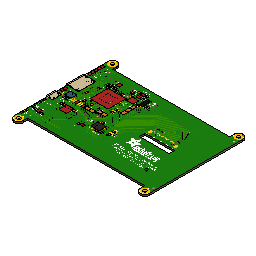
Adafruit 5in HDMI Backpack v2 (Autodesk Fusion 360 design; units mm, degrees)
part number: 47151-0001
part number: TFP401
part number: 1uF
part number: Ferrite
part number: MOUNTINGHOLE3.0
part number: FIDUCIAL""
part number: FAN5333BSX
part number: LT1117(3V3)
part number: MicroUSB
part number: AR1100
part number: 12MHz
part number: 33
part number: Blue
part number: 15uH
part number: MBR0540
part number: MM3Z24VT1G
part number: BSS138
part number: TFTLCD-KD50G21-40NT-A1
part number: 1N4148
part number: 100uF/6V
Autodesk Fusion 360 part; units mm, degrees
sketch "sketch 301" plane through (0, 0, 0) normal (0, 0, 1) x (1, 0, 0)
  line L0 (8, 0) -> (112.7, 0)
  line L1 (112.7, 0) -> (112.7, -4)
  arc A0 (112.7, -4) -> (116.7, -8) centre (116.7, -4) ccw
  arc A1 (116.7, -8) -> (120.7, -4) centre (116.7, -4) ccw
  line L2 (120.7, -4) -> (120.7, 79.8)
  arc A2 (120.7, 79.8) -> (116.7, 83.8) centre (116.7, 79.8) ccw
  arc A3 (116.7, 83.8) -> (112.7, 79.9) centre (116.65, 79.85) ccw
  line L3 (112.7, 79.9) -> (112.7, 75.8)
  line L4 (112.7, 75.8) -> (8, 75.8)
  line L5 (8, 75.8) -> (8, 79.8)
  arc A4 (8, 79.8) -> (4, 83.8) centre (4, 79.8) ccw
  arc A5 (4, 83.8) -> (0, 79.8) centre (4, 79.8) ccw
  line L6 (0, 79.8) -> (0, -4)
  arc A6 (0, -4) -> (4, -8) centre (4, -4) ccw
  arc A7 (4, -8) -> (8, -4) centre (4, -4) ccw
  line L7 (8, -4) -> (8, 0)
  line L8 (98.778, 35.73) -> (98.778, 40.752)
  line L9 (98.778, 40.752) -> (72.108, 40.752)
  line L10 (72.108, 40.752) -> (72.108, 35.73)
  line L11 (72.108, 35.73) -> (98.778, 35.73)
  arc A8 (7.15, 58.25) -> (7.6, 57.8) centre (7.6, 58.25) ccw
  arc A9 (7.6, 58.7) -> (7.15, 58.25) centre (7.6, 58.25) ccw
  line L12 (7.6, 58.7) -> (9.4, 58.7)
  arc A10 (9.85, 58.25) -> (9.4, 58.7) centre (9.4, 58.25) ccw
  arc A11 (9.4, 57.8) -> (9.85, 58.25) centre (9.4, 58.25) ccw
  line L13 (9.4, 57.8) -> (7.6, 57.8)
  arc A12 (2.13, 44.2) -> (1.68, 43.75) centre (2.13, 43.75) ccw
  line L14 (2.13, 44.2) -> (2.93, 44.2)
  arc A13 (3.38, 43.75) -> (2.93, 44.2) centre (2.93, 43.75) ccw
  arc A14 (2.93, 43.3) -> (3.38, 43.75) centre (2.93, 43.75) ccw
  line L15 (2.93, 43.3) -> (2.13, 43.3)
  arc A15 (1.68, 43.75) -> (2.13, 43.3) centre (2.13, 43.75) ccw
  line L16 (7.6, 43.3) -> (9.4, 43.3)
  arc A16 (9.4, 43.3) -> (9.85, 43.75) centre (9.4, 43.75) ccw
  arc A17 (9.85, 43.75) -> (9.4, 44.2) centre (9.4, 43.75) ccw
  line L17 (9.4, 44.2) -> (7.6, 44.2)
  arc A18 (7.6, 44.2) -> (7.15, 43.75) centre (7.6, 43.75) ccw
  arc A19 (7.15, 43.75) -> (7.6, 43.3) centre (7.6, 43.75) ccw
  arc A20 (2.13, 58.7) -> (1.68, 58.25) centre (2.13, 58.25) ccw
  line L18 (2.13, 58.7) -> (2.93, 58.7)
  arc A21 (3.38, 58.25) -> (2.93, 58.7) centre (2.93, 58.25) ccw
  arc A22 (2.93, 57.8) -> (3.38, 58.25) centre (2.93, 58.25) ccw
  line L19 (2.93, 57.8) -> (2.13, 57.8)
  arc A23 (1.68, 58.25) -> (2.13, 57.8) centre (2.13, 58.25) ccw
  arc A24 (2.4, 33.2) -> (2.15, 33.5) centre (2.125, 33.225) ccw
  arc A25 (2.15, 32.9) -> (2.4, 33.2) centre (2.125, 33.175) ccw
  line L20 (2.15, 32.9) -> (1.55, 32.9)
  arc A26 (1.3, 33.2) -> (1.55, 32.9) centre (1.575, 33.175) ccw
  arc A27 (1.55, 33.5) -> (1.3, 33.2) centre (1.575, 33.225) ccw
  line L21 (1.55, 33.5) -> (2.15, 33.5)
  arc A28 (2.15, 25.7) -> (2.4, 26) centre (2.125, 25.975) ccw
  line L22 (2.15, 25.7) -> (1.55, 25.7)
  arc A29 (1.3, 26) -> (1.55, 25.7) centre (1.575, 25.975) ccw
  arc A30 (1.55, 26.3) -> (1.3, 26) centre (1.575, 26.025) ccw
  line L23 (1.55, 26.3) -> (2.15, 26.3)
  arc A31 (2.4, 26) -> (2.15, 26.3) centre (2.125, 26.025) ccw
extrude "Board" add sketch "sketch 301" along normal blind 1.57 makes body 1 in component "Board"
sketch "sketch 2066" plane through (0, 0, 0) normal (0, 0, 1) x (1, 0, 0)
  line L0 (-7.7, -10.31) -> (7.7, -10.31)
  line L1 (7.7, -10.31) -> (7.7, 1)
  line L2 (7.7, 1) -> (-7.7, 1)
  line L3 (-7.7, 1) -> (-7.7, -10.31)
extrude "HDMI_MOLEX_47151-0001_DIMLAYER" add sketch "sketch 2066" along normal blind 0.1 separate body makes body 2 in component "HDMI_MOLEX_47151-0001_DIMLAYER"
sketch "sketch 2197" plane through (0, 0, 0) normal (0, 0, 1) x (1, 0, 0)
  line L0 (-8.12, -8.12) -> (8, -8.12)
  line L1 (8, -8.12) -> (8, 8)
  line L2 (8, 8) -> (-8.12, 8)
  line L3 (-8.12, 8) -> (-8.12, -8.12)
extrude "S-PQFP-G100" add sketch "sketch 2197" along normal blind 0.1 separate body makes body 3 in component "S-PQFP-G100"
sketch "sketch 2584" plane through (0, 0, 0) normal (0, 0, 1) x (1, 0, 0)
  line L0 (-1.092, -0.724) -> (1.106, -0.724)
  line L1 (1.106, -0.724) -> (1.106, 0.726)
  line L2 (1.106, 0.726) -> (-1.092, 0.726)
  line L3 (-1.092, 0.726) -> (-1.092, -0.724)
extrude "0805-NO" add sketch "sketch 2584" along normal blind 0.1 separate body makes body 4 in component "0805-NO"
sketch "sketch 2803" plane through (0, 0, 0) normal (0, 0, 1) x (1, 0, 0)
  line L0 (-1, -0.65) -> (1, -0.65)
  line L1 (1, -0.65) -> (1, 0.65)
  line L2 (1, 0.65) -> (-1, 0.65)
  line L3 (-1, 0.65) -> (-1, -0.65)
extrude "_0805MP" add sketch "sketch 2803" along normal blind 0.1 separate body makes body 5 in component "_0805MP"
sketch "sketch 2942" plane through (0, 0, 0) normal (0, 0, 1) x (1, 0, 0)
  line L0 (-1.651, -1.016) -> (1.651, -1.016)
  line L1 (1.651, -1.016) -> (1.651, 1.016)
  line L2 (1.651, 1.016) -> (-1.651, 1.016)
  line L3 (-1.651, 1.016) -> (-1.651, -1.016)
extrude "SOLDERJUMPER_ARROW_NOPASTE" add sketch "sketch 2942" along normal blind 0.1 separate body makes body 6 in component "SOLDERJUMPER_ARROW_NOPASTE"
sketch "sketch 3097" plane through (0, 0, 0) normal (0, 0, 1) x (1, 0, 0)
  line L0 (-3.429, -3.429) -> (3.429, -3.429)
  line L1 (3.429, -3.429) -> (3.429, 3.429)
  line L2 (3.429, 3.429) -> (-3.429, 3.429)
  line L3 (-3.429, 3.429) -> (-3.429, -3.429)
extrude "MOUNTINGHOLE_3.0_PLATED" add sketch "sketch 3097" along normal blind 0.1 separate body makes body 7 in component "MOUNTINGHOLE_3.0_PLATED"
sketch "sketch 3268" plane through (0, 0, 0) normal (0, 0, 1) x (1, 0, 0)
  line L0 (-0.75, -0.75) -> (0.75, -0.75)
  line L1 (0.75, -0.75) -> (0.75, 0.75)
  line L2 (0.75, 0.75) -> (-0.75, 0.75)
  line L3 (-0.75, 0.75) -> (-0.75, -0.75)
extrude "FIDUCIAL_1MM" add sketch "sketch 3268" along normal blind 0.1 separate body makes body 8 in component "FIDUCIAL_1MM"
sketch "sketch 3407" plane through (0, 0, 0) normal (0, 0, 1) x (1, 0, 0)
  line L0 (-1.65, -1.5) -> (1.65, -1.5)
  line L1 (1.65, -1.5) -> (1.65, 1.5)
  line L2 (1.65, 1.5) -> (-1.65, 1.5)
  line L3 (-1.65, 1.5) -> (-1.65, -1.5)
extrude "SOT23-5" add sketch "sketch 3407" along normal blind 0.1 separate body makes body 9 in component "SOT23-5"
sketch "sketch 3538" plane through (0, 0, 0) normal (0, 0, 1) x (1, 0, 0)
  line L0 (-3.35, -3.45) -> (3.35, -3.45)
  line L1 (3.35, -3.45) -> (3.35, 3.45)
  line L2 (3.35, 3.45) -> (-3.35, 3.45)
  line L3 (-3.35, 3.45) -> (-3.35, -3.45)
extrude "SOT223-R" add sketch "sketch 3538" along normal blind 0.1 separate body makes body 10 in component "SOT223-R"
sketch "sketch 3669" plane through (0, 0, 0) normal (0, 0, 1) x (1, 0, 0)
  line L0 (-3.975, -4.9) -> (4.35, -4.9)
  line L1 (4.35, -4.9) -> (4.35, 1.25)
  line L2 (4.35, 1.25) -> (-3.975, 1.25)
  line L3 (-3.975, 1.25) -> (-3.975, -4.9)
extrude "4UCONN_20329" add sketch "sketch 3669" along normal blind 0.1 separate body makes body 11 in component "4UCONN_20329"
sketch "sketch 3800" plane through (0, 0, 0) normal (0, 0, 1) x (1, 0, 0)
  line L0 (-3.165, -3.821) -> (3.165, -3.821)
  line L1 (3.165, -3.821) -> (3.165, 3.821)
  line L2 (3.165, 3.821) -> (-3.165, 3.821)
  line L3 (-3.165, 3.821) -> (-3.165, -3.821)
extrude "TSSOP20-5.3MMBODY" add sketch "sketch 3800" along normal blind 0.1 separate body makes body 12 in component "TSSOP20-5.3MMBODY"
sketch "sketch 3931" plane through (0, 0, 0) normal (0, 0, 1) x (1, 0, 0)
  line L0 (-1.8, -0.65) -> (1.8, -0.65)
  line L1 (1.8, -0.65) -> (1.8, 0.65)
  line L2 (1.8, 0.65) -> (-1.8, 0.65)
  line L3 (-1.8, 0.65) -> (-1.8, -0.65)
extrude "RESONATOR-SMD" add sketch "sketch 3931" along normal blind 0.1 separate body makes body 13 in component "RESONATOR-SMD"
sketch "sketch 4110" plane through (0, 0, 0) normal (0, 0, 1) x (1, 0, 0)
  line L0 (-1.9, -1.4) -> (1.9, -1.4)
  line L1 (1.9, -1.4) -> (1.9, 1.4)
  line L2 (1.9, 1.4) -> (-1.9, 1.4)
  line L3 (-1.9, 1.4) -> (-1.9, -1.4)
extrude "RESPACK_4X0603" add sketch "sketch 4110" along normal blind 0.1 separate body makes body 14 in component "RESPACK_4X0603"
sketch "sketch 4257" plane through (0, 0, 0) normal (0, 0, 1) x (1, 0, 0)
  line L0 (-0.625, -1.3334) -> (0.625, -1.3334)
  line L1 (0.625, -1.3334) -> (0.625, 1.3334)
  line L2 (0.625, 1.3334) -> (-0.625, 1.3334)
  line L3 (-0.625, 1.3334) -> (-0.625, -1.3334)
extrude "CHIPLED_0805_NOOUTLINE" add sketch "sketch 4257" along normal blind 0.1 separate body makes body 15 in component "CHIPLED_0805_NOOUTLINE"
sketch "sketch 4388" plane through (0, 0, 0) normal (0, 0, 1) x (1, 0, 0)
  line L0 (-2.938, -2.6) -> (2.938, -2.6)
  line L1 (2.938, -2.6) -> (2.938, 2.6)
  line L2 (2.938, 2.6) -> (-2.938, 2.6)
  line L3 (-2.938, 2.6) -> (-2.938, -2.6)
extrude "INDUCTOR_5X5MM_NR5040_NOTHERMALS" add sketch "sketch 4388" along normal blind 0.1 separate body makes body 16 in component "INDUCTOR_5X5MM_NR5040_NOTHERMALS"
sketch "sketch 4519" plane through (0, 0, 0) normal (0, 0, 1) x (1, 0, 0)
  line L0 (-1.723, -0.7) -> (1.723, -0.7)
  line L1 (1.723, -0.7) -> (1.723, 0.7)
  line L2 (1.723, 0.7) -> (-1.723, 0.7)
  line L3 (-1.723, 0.7) -> (-1.723, -0.7)
extrude "SOD-123" add sketch "sketch 4519" along normal blind 0.1 separate body makes body 17 in component "SOD-123"
sketch "sketch 4650" plane through (0, 0, 0) normal (0, 0, 1) x (1, 0, 0)
  line L0 (-3.889, -1.6) -> (3.916, -1.6)
  line L1 (3.916, -1.6) -> (3.916, 1.6)
  line L2 (3.916, 1.6) -> (-3.889, 1.6)
  line L3 (-3.889, 1.6) -> (-3.889, -1.6)
extrude "SMADIODE" add sketch "sketch 4650" along normal blind 0.1 separate body makes body 18 in component "SMADIODE"
sketch "sketch 4781" plane through (0, 0, 0) normal (0, 0, 1) x (1, 0, 0)
  line L0 (-1.672, -1.295) -> (1.672, -1.295)
  line L1 (1.672, -1.295) -> (1.672, 1.295)
  line L2 (1.672, 1.295) -> (-1.672, 1.295)
  line L3 (-1.672, 1.295) -> (-1.672, -1.295)
extrude "SOT23-WIDE" add sketch "sketch 4781" along normal blind 0.1 separate body makes body 19 in component "SOT23-WIDE"
sketch "sketch 4912" plane through (0, 0, 0) normal (0, 0, 1) x (1, 0, 0)
  line L0 (0, 0) -> (120.7, 0)
  line L1 (120.7, 0) -> (120.7, 75.8)
  line L2 (120.7, 75.8) -> (0, 75.8)
  line L3 (0, 75.8) -> (0, 0)
extrude "TFTLCD-KD50G21-40NT-A1" add sketch "sketch 4912" along normal blind 0.1 separate body makes body 20 in component "TFTLCD-KD50G21-40NT-A1"
sketch "sketch 5091" plane through (0, 0, 0) normal (0, 0, 1) x (1, 0, 0)
  line L0 (-1.2, -1.2) -> (1.2, -1.2)
  line L1 (1.2, -1.2) -> (1.2, 1.2)
  line L2 (1.2, 1.2) -> (-1.2, 1.2)
  line L3 (-1.2, 1.2) -> (-1.2, -1.2)
extrude "1X01_SMD_MASKHELD_2X2MM" add sketch "sketch 5091" along normal blind 0.1 separate body makes body 21 in component "1X01_SMD_MASKHELD_2X2MM"
sketch "sketch 5230" plane through (0, 0, 0) normal (0, 0, 1) x (1, 0, 0)
  line L0 (-1.651, -1.016) -> (1.651, -1.016)
  line L1 (1.651, -1.016) -> (1.651, 1.016)
  line L2 (1.651, 1.016) -> (-1.651, 1.016)
  line L3 (-1.651, 1.016) -> (-1.651, -1.016)
extrude "SOLDERJUMPER_CLOSEDWIRE" add sketch "sketch 5230" along normal blind 0.1 separate body makes body 22 in component "SOLDERJUMPER_CLOSEDWIRE"
sketch "sketch 5361" plane through (0, 0, 0) normal (0, 0, 1) x (1, 0, 0)
  line L0 (-1, -0.7) -> (1, -0.7)
  line L1 (1, -0.7) -> (1, 0.7)
  line L2 (1, 0.7) -> (-1, 0.7)
  line L3 (-1, 0.7) -> (-1, -0.7)
extrude "SOD-323" add sketch "sketch 5361" along normal blind 0.1 separate body makes body 23 in component "SOD-323"
sketch "sketch 5492" plane through (0, 0, 0) normal (0, 0, 1) x (1, 0, 0)
  line L0 (-2.95, -2.6) -> (2.95, -2.6)
  line L1 (2.95, -2.6) -> (2.95, 2.6)
  line L2 (2.95, 2.6) -> (-2.95, 2.6)
  line L3 (-2.95, 2.6) -> (-2.95, -2.6)
extrude "PANASONIC_C" add sketch "sketch 5492" along normal blind 0.1 separate body makes body 24 in component "PANASONIC_C"
sketch "sketch 5623" plane through (0, 0, 0) normal (0, 0, 1) x (1, 0, 0)
  line L0 (0.241, -0.013) -> (29.654, -0.013)
  line L1 (29.654, -0.013) -> (29.654, 11.544)
  line L2 (29.654, 11.544) -> (0.241, 11.544)
  line L3 (0.241, 11.544) -> (0.241, -0.013)
extrude "ADAFRUIT_TEXT_30MM" add sketch "sketch 5623" along normal blind 0.1 separate body makes body 25 in component "ADAFRUIT_TEXT_30MM"
sketch "sketch 5754" plane through (0, 0, 0) normal (0, 0, 1) x (1, 0, 0)
  line L0 (-1.092, -1.092) -> (1.092, -1.092)
  line L1 (1.092, -1.092) -> (1.092, 1.092)
  line L2 (1.092, 1.092) -> (-1.092, 1.092)
  line L3 (-1.092, 1.092) -> (-1.092, -1.092)
extrude "PCBFEAT-REV-056" add sketch "sketch 5754" along normal blind 0.1 separate body makes body 26 in component "PCBFEAT-REV-056"
sketch "sketch 707" plane through (0, 0, 0) normal (0, 0, 1) x (1, 0, 0)
  circle A0 centre (21.15, 57.85) radius 0.2
  circle A1 centre (38.8, 42.4) radius 0.2
  circle A2 centre (43.75, 46) radius 0.2
  circle A3 centre (38.8, 44.25) radius 0.2
  circle A4 centre (38.25, 52.65) radius 0.2
  circle A5 centre (42.2, 54.9) radius 0.2
  circle A6 centre (6.15, 54.5) radius 0.2
  circle A7 centre (14.5, 43.75) radius 0.2
  circle A8 centre (7.5, 45.85) radius 0.2
  circle A9 centre (9.45, 38.65) radius 0.2
  circle A10 centre (18.523, 37) radius 0.2
  circle A11 centre (32.3, 40.05) radius 0.2
  circle A12 centre (8.5, 56.6) radius 0.2
  circle A13 centre (20.7, 25.8) radius 0.2
  circle A14 centre (25.015, 36.7) radius 0.2
  circle A15 centre (22.6, 41.8) radius 0.2
  circle A16 centre (41.4, 66.5) radius 0.2
  circle A17 centre (20.9, 66.5) radius 0.2
  circle A18 centre (19.05, 56.2) radius 0.2
  circle A19 centre (29.45, 60.35) radius 0.2
  circle A20 centre (17.196, 31.25) radius 0.2
  circle A21 centre (12.099, 31.692) radius 0.2
  circle A22 centre (24.981, 31.211) radius 0.2
  circle A23 centre (12.376, 28.65) radius 0.2
  circle A24 centre (19.25, 67.95) radius 0.2
  circle A25 centre (10.65, 67.35) radius 0.2
  circle A26 centre (34, 63.6) radius 0.2
  circle A27 centre (35.8, 68.6) radius 0.2
  circle A28 centre (19.684, 28.573) radius 0.2
  circle A29 centre (45, 57.6) radius 0.2
  circle A30 centre (38.4, 57.5) radius 0.2
  circle A31 centre (26.867, 22.731) radius 0.2
  circle A32 centre (26.997, 26.801) radius 0.2
  circle A33 centre (34.55, 28.396) radius 0.2
  circle A34 centre (17.144, 24.911) radius 0.2
  circle A35 centre (80.258, 49.98) radius 0.2
  circle A36 centre (77.435, 44.606) radius 0.2
  circle A37 centre (93.308, 48.93) radius 0.2
  circle A38 centre (93.812, 44.66) radius 0.2
  circle A39 centre (75.158, 49.23) radius 0.2
  circle A40 centre (35.65, 26.396) radius 0.2
  circle A41 centre (36.75, 22.096) radius 0.2
  circle A42 centre (40.25, 51.5) radius 0.2
  circle A43 centre (1.067, 15.331) radius 0.2
  circle A44 centre (3.5, 64.9) radius 0.2
  circle A45 centre (24.667, 22.731) radius 0.2
  circle A46 centre (24.667, 24.931) radius 0.2
  circle A47 centre (26.867, 24.931) radius 0.2
  circle A48 centre (24.767, 20.031) radius 0.2
  circle A49 centre (26.767, 20.031) radius 0.2
  circle A50 centre (26.767, 18.231) radius 0.2
  circle A51 centre (24.767, 18.231) radius 0.2
  circle A52 centre (28.762, 29.79) radius 0.2
  circle A53 centre (13.967, 22.331) radius 0.2
  circle A54 centre (13.967, 19.931) radius 0.2
  circle A55 centre (19.167, 8.331) radius 0.2
  circle A56 centre (19.167, 11.131) radius 0.2
  circle A57 centre (19.167, 4.531) radius 0.2
  circle A58 centre (33.8, 67.9) radius 0.2
  circle A59 centre (36.848, 66.503) radius 0.2
  circle A60 centre (33.673, 66.122) radius 0.2
  circle A61 centre (19.482, 31.25) radius 0.2
  circle A62 centre (22.784, 32.266) radius 0.2
  circle A63 centre (7.146, 31.946) radius 0.2
  circle A64 centre (17.5, 52.75) radius 0.2
  circle A65 centre (13, 52.75) radius 0.2
  circle A66 centre (13, 51.5) radius 0.2
  circle A67 centre (17.5, 51.5) radius 0.2
  circle A68 centre (16, 55.75) radius 0.2
  circle A69 centre (18, 55.7) radius 0.2
  circle A70 centre (16, 54.5) radius 0.2
  circle A71 centre (17.5, 54.5) radius 0.2
  circle A72 centre (31.9, 38.95) radius 0.2
  circle A73 centre (36.2, 28.5) radius 0.2
  circle A74 centre (18.4, 25.75) radius 0.2
  circle A75 centre (18.4, 32.1) radius 0.2
  circle A76 centre (92.458, 43.898) radius 0.2
  circle A77 centre (3.7, 38.3) radius 0.2
  circle A78 centre (5.886, 21.15) radius 0.2
  circle A79 centre (34.798, 21.336) radius 0.25
  circle A80 centre (38.85, 51.35) radius 0.2
  circle A81 centre (24.746, 39.154) radius 0.2
  circle A82 centre (29.6, 62.1) radius 0.2
  circle A83 centre (21.25, 42) radius 0.2
  circle A84 centre (22.1, 37.7) radius 0.2
  circle A85 centre (23.6, 41.004) radius 0.2
  circle A86 centre (23.7, 37.7) radius 0.2
  circle A87 centre (12.9, 43.75) radius 0.2
  circle A88 centre (13.171, 38.55) radius 0.2
  circle A89 centre (19.9, 64.35) radius 0.2
  circle A90 centre (5.4, 67.7) radius 0.2
  circle A91 centre (22.1, 64.45) radius 0.2
  circle A92 centre (6.4, 70.5) radius 0.2
  circle A93 centre (6.909, 35.25) radius 0.2
  circle A94 centre (39.7, 63.6) radius 0.2
  circle A95 centre (35.3, 63.6) radius 0.2
  circle A96 centre (37.7, 58.7) radius 0.2
  circle A97 centre (16.002, 25.4) radius 0.25
  circle A98 centre (6.9, 55.6) radius 0.2
  circle A99 centre (17.5, 59.4) radius 0.2
  circle A100 centre (3.6, 62.1) radius 0.2
  circle A101 centre (93.408, 52.88) radius 0.2
  circle A102 centre (94.508, 53.98) radius 0.2
  circle A103 centre (92.608, 53.68) radius 0.2
  circle A104 centre (94.058, 55.13) radius 0.2
  circle A105 centre (91.758, 54.53) radius 0.2
  circle A106 centre (93.558, 56.33) radius 0.2
  circle A107 centre (90.908, 55.38) radius 0.2
  circle A108 centre (93.058, 57.53) radius 0.2
  circle A109 centre (90.058, 56.23) radius 0.2
  circle A110 centre (92.558, 58.73) radius 0.2
  circle A111 centre (89.208, 57.08) radius 0.2
  circle A112 centre (92.058, 59.93) radius 0.2
  circle A113 centre (88.358, 57.93) radius 0.2
  circle A114 centre (91.558, 61.13) radius 0.2
  circle A115 centre (44.75, 44.7) radius 0.2
  circle A116 centre (34.1, 35) radius 0.2
  circle A117 centre (45.75, 43.9) radius 0.2
  circle A118 centre (34.95, 34.2) radius 0.2
  circle A119 centre (46.65, 43.1) radius 0.2
  circle A120 centre (35.8, 35) radius 0.2
  circle A121 centre (47.55, 42.3) radius 0.2
  circle A122 centre (36.9, 34.15) radius 0.2
  circle A123 centre (48.45, 41.5) radius 0.2
  circle A124 centre (38.2, 35) radius 0.2
  circle A125 centre (49.35, 40.7) radius 0.2
  circle A126 centre (39.05, 34.15) radius 0.2
  circle A127 centre (50.25, 39.9) radius 0.2
  circle A128 centre (39.9, 35) radius 0.2
  circle A129 centre (51.15, 39.1) radius 0.2
  circle A130 centre (40.75, 34.15) radius 0.2
  circle A131 centre (25.9, 32.2) radius 0.2
  circle A132 centre (45.35, 38.3) radius 0.2
  circle A133 centre (26.75, 31.15) radius 0.2
  circle A134 centre (46.25, 37.5) radius 0.2
  circle A135 centre (27.6, 32.2) radius 0.2
  circle A136 centre (47.15, 36.7) radius 0.2
  circle A137 centre (28.45, 31.15) radius 0.2
  circle A138 centre (48.05, 35.9) radius 0.2
  circle A139 centre (29.75, 30.95) radius 0.2
  circle A140 centre (48.95, 35.1) radius 0.2
  circle A141 centre (31.05, 30.45) radius 0.2
  circle A142 centre (49.85, 34.3) radius 0.2
  circle A143 centre (32.35, 29.85) radius 0.2
  circle A144 centre (50.75, 33.5) radius 0.2
  circle A145 centre (33.65, 29.25) radius 0.2
  circle A146 centre (51.65, 32.7) radius 0.2
  circle A147 centre (78.566, 44.06) radius 0.2
  circle A148 centre (51.2, 55.7) radius 0.2
  circle A149 centre (77.708, 49.53) radius 0.2
  circle A150 centre (52.1, 56.6) radius 0.2
  circle A151 centre (79.208, 49.53) radius 0.2
  circle A152 centre (53.4, 54) radius 0.2
  circle A153 centre (76.208, 49.53) radius 0.2
  circle A154 centre (50.3, 54.9) radius 0.2
  circle A155 centre (26.65, 41.65) radius 0.2
  circle A156 centre (25.802, 25.901) radius 0.2
  circle A157 centre (79.548, 44.568) radius 0.2
  circle A158 centre (56.462, 67.7) radius 0.2
  circle A159 centre (51.816, 26.841) radius 0.2
  circle A160 centre (60.841, 26.841) radius 0.2
  circle A161 centre (44.877, 25.31) radius 0.2
  circle A162 centre (60, 25.31) radius 0.2
  circle A163 centre (45.158, 23.642) radius 0.2
  circle A164 centre (56.299, 22.02) radius 0.2
  circle A165 centre (38.65, 67.35) radius 0.2
  circle A166 centre (50.946, 67.7) radius 0.2
  circle A167 centre (56.3, 60.1) radius 0.2
  circle A168 centre (95.708, 47.93) radius 0.2
  circle A169 centre (52.9, 59.2) radius 0.2
  circle A170 centre (94.348, 48.87) radius 0.2
  circle A171 centre (46.164, 21.821) radius 0.2
  circle A172 centre (51.5, 28.7) radius 0.2
  circle A173 centre (50.945, 20.09) radius 0.2
  circle A174 centre (40.512, 26.452) radius 0.2
  circle A175 centre (57.314, 22.614) radius 0.2
  circle A176 centre (53.714, 22.414) radius 0.2
  circle A177 centre (40.712, 21.952) radius 0.2
  circle A178 centre (8.49, 58.25) radius 0.45
  circle A179 centre (8.49, 43.75) radius 0.45
  circle A180 centre (2.53, 43.75) radius 0.45
  circle A181 centre (2.53, 58.25) radius 0.45
  circle A182 centre (25, 55) radius 0.2
  circle A183 centre (27, 55) radius 0.2
  circle A184 centre (29, 55) radius 0.2
  circle A185 centre (31, 55) radius 0.2
  circle A186 centre (33, 55) radius 0.2
  circle A187 centre (33, 53) radius 0.2
  circle A188 centre (33, 51) radius 0.2
  circle A189 centre (33, 49) radius 0.2
  circle A190 centre (33, 47) radius 0.2
  circle A191 centre (31, 47) radius 0.2
  circle A192 centre (29, 47) radius 0.2
  circle A193 centre (27, 47) radius 0.2
  circle A194 centre (25, 47) radius 0.2
  circle A195 centre (25, 49) radius 0.2
  circle A196 centre (25, 51) radius 0.2
  circle A197 centre (25, 53) radius 0.2
  circle A198 centre (4, 79.8) radius 1.5
  circle A199 centre (116.7, 79.8) radius 1.5
  circle A200 centre (116.7, -4) radius 1.5
  circle A201 centre (4, -4) radius 1.5
  circle A202 centre (3.75, 31.55) radius 0.35
  circle A203 centre (3.75, 27.65) radius 0.35
  circle A204 centre (1.85, 26) radius 0.3
  circle A205 centre (1.85, 33.2) radius 0.3
  circle A206 centre (4.65, 32.9) radius 0.35
  circle A207 centre (4.65, 26.3) radius 0.35
extrude "Extrude2" cut sketch "sketch 707" along normal blind 1.57 bodies 1 in component "Board"
component "PCB Component" placed x (1, 0, 0) y (0, 1, 0) z (0, 0, 1) at (0, 0, 0)
component "Board" placed x (1, 0, 0) y (0, 1, 0) z (0, 0, 1) at (0, 0, 0) in component "PCB Component"
component "HDMI_MOLEX_47151-0001_DIMLAYER" placed x (0, -1, 0) y (1, 0, 0) z (0, 0, 1) at (9.25, 51, 1.57) in component "PCB Component"
component "S-PQFP-G100" placed x (1, 0, 0) y (0, 1, 0) z (0, 0, 1) at (29, 51, 1.57) in component "PCB Component"
component "0805-NO" placed x (0, -1, 0) y (1, 0, 0) z (0, 0, 1) at (17.7, 61.9, 1.57) in component "PCB Component"
component "0805-NO" placed x (0, -1, 0) y (1, 0, 0) z (0, 0, 1) at (26.3, 39, 1.57) in component "PCB Component"
component "0805-NO" placed x (-1, 0, 0) y (0, -1, 0) z (0, 0, 1) at (27.05, 60.8, 1.57) in component "PCB Component"
component "0805-NO" placed x (1, 0, 0) y (0, 1, 0) z (0, 0, 1) at (41.2, 45.873, 1.57) in component "PCB Component"
component "0805-NO" placed x (-1, 0, 0) y (0, -1, 0) z (0, 0, 1) at (31.75, 60.8, 1.57) in component "PCB Component"
component "0805-NO" placed x (1, 0, 0) y (0, 1, 0) z (0, 0, 1) at (20.25, 59.25, 1.57) in component "PCB Component"
component "0805-NO" placed x (0, -1, 0) y (1, 0, 0) z (0, 0, 1) at (10.509, 32.772, 1.57) in component "PCB Component"
component "0805-NO" placed x (0, -1, 0) y (1, 0, 0) z (0, 0, 1) at (20, 38.75, 1.57) in component "PCB Component"
component "0805-NO" placed x (0, -1, 0) y (1, 0, 0) z (0, 0, 1) at (14.5, 46.25, 1.57) in component "PCB Component"
component "0805-NO" placed x (0, -1, 0) y (1, 0, 0) z (0, 0, 1) at (19.9, 61.9, 1.57) in component "PCB Component"
component "0805-NO" placed x (0, -1, 0) y (1, 0, 0) z (0, 0, 1) at (22.1, 61.9, 1.57) in component "PCB Component"
component "0805-NO" placed x (0, -1, 0) y (1, 0, 0) z (0, 0, 1) at (8.609, 32.772, 1.57) in component "PCB Component"
component "0805-NO" placed x (0, 1, 0) y (-1, 0, 0) z (0, 0, 1) at (13.9, 26.3, 1.57) in component "PCB Component"
component "0805-NO" placed x (0, 1, 0) y (-1, 0, 0) z (0, 0, 1) at (22.9, 26.3, 1.57) in component "PCB Component"
component "0805-NO" placed x (-1, 0, 0) y (0, -1, 0) z (0, 0, 1) at (41.2, 42.4, 1.57) in component "PCB Component"
component "0805-NO" placed x (1, 0, 0) y (0, 1, 0) z (0, 0, 1) at (48.641, 20.821, 1.57) in component "PCB Component"
component "0805-NO" placed x (-1, 0, 0) y (0, -1, 0) z (0, 0, 1) at (45.441, 29.811, 1.57) in component "PCB Component"
component "0805-NO" placed x (0, 1, 0) y (-1, 0, 0) z (0, 0, 1) at (1.223, 5.882, 1.57) in component "PCB Component"
component "0805-NO" placed x (0, -1, 0) y (1, 0, 0) z (0, 0, 1) at (37.65, 64.2, 1.57) in component "PCB Component"
component "0805-NO" placed x (0, 1, 0) y (-1, 0, 0) z (0, 0, 1) at (54, 61.5, 1.57) in component "PCB Component"
component "0805-NO" placed x (0, 1, 0) y (-1, 0, 0) z (0, 0, 1) at (51.8, 61.5, 1.57) in component "PCB Component"
component "0805-NO" placed x (0, -1, 0) y (1, 0, 0) z (0, 0, 1) at (45, 66.1, 1.57) in component "PCB Component"
component "0805-NO" placed x (0, 1, 0) y (-1, 0, 0) z (0, 0, 1) at (44.954, 69.728, 1.57) in component "PCB Component"
component "0805-NO" placed x (0, 1, 0) y (-1, 0, 0) z (0, 0, 1) at (35.3, 66.1, 1.57) in component "PCB Component"
component "0805-NO" placed x (0, -1, 0) y (1, 0, 0) z (0, 0, 1) at (24.3, 61.9, 1.57) in component "PCB Component"
component "0805-NO" placed x (0, -1, 0) y (1, 0, 0) z (0, 0, 1) at (1.1, 17.7, 1.57) in component "PCB Component"
component "0805-NO" placed x (1, 0, 0) y (0, 1, 0) z (0, 0, 1) at (3.678, 10.698, 1.57) in component "PCB Component"
component "0805-NO" placed x (-1, 0, 0) y (0, -1, 0) z (0, 0, 1) at (10.957, 9.771, 1.57) in component "PCB Component"
component "0805-NO" placed x (-1, 0, 0) y (0, -1, 0) z (0, 0, 1) at (57.315, 27.735, 1.57) in component "PCB Component"
component "0805-NO" placed x (1, 0, 0) y (0, 1, 0) z (0, 0, 1) at (57.315, 23.925, 1.57) in component "PCB Component"
component "0805-NO" placed x (0, -1, 0) y (1, 0, 0) z (0, 0, 1) at (34.983, 18.473, 1.57) in component "PCB Component"
component "0805-NO" placed x (-1, 0, 0) y (0, -1, 0) z (0, 0, 1) at (38.227, 69.596, 1.57) in component "PCB Component"
component "0805-NO" placed x (0, 1, 0) y (-1, 0, 0) z (0, 0, 1) at (11.684, 26.416, 1.57) in component "PCB Component"
component "_0805MP" placed x (0, 1, 0) y (-1, 0, 0) z (0, 0, 1) at (15.882, 34.55, 1.57) in component "PCB Component"
component "_0805MP" placed x (-1, 0, 0) y (0, -1, 0) z (0, 0, 1) at (41.2, 44.073, 1.57) in component "PCB Component"
component "_0805MP" placed x (0, 1, 0) y (-1, 0, 0) z (0, 0, 1) at (12.536, 34.55, 1.57) in component "PCB Component"
component "_0805MP" placed x (0, 1, 0) y (-1, 0, 0) z (0, 0, 1) at (14.209, 34.55, 1.57) in component "PCB Component"
component "_0805MP" placed x (0, 1, 0) y (-1, 0, 0) z (0, 0, 1) at (40.8, 54, 1.57) in component "PCB Component"
component "_0805MP" placed x (0, -1, 0) y (1, 0, 0) z (0, 0, 1) at (19.915, 34.411, 1.57) in component "PCB Component"
component "_0805MP" placed x (0, 1, 0) y (-1, 0, 0) z (0, 0, 1) at (21.619, 34.423, 1.57) in component "PCB Component"
component "_0805MP" placed x (1, 0, 0) y (0, 1, 0) z (0, 0, 1) at (43.561, 20.821, 1.57) in component "PCB Component"
component "_0805MP" placed x (1, 0, 0) y (0, 1, 0) z (0, 0, 1) at (57.315, 29.64, 1.57) in component "PCB Component"
component "_0805MP" placed x (1, 0, 0) y (0, 1, 0) z (0, 0, 1) at (57.315, 25.83, 1.57) in component "PCB Component"
component "_0805MP" placed x (-1, 0, 0) y (0, -1, 0) z (0, 0, 1) at (48.641, 18.843, 1.57) in component "PCB Component"
component "_0805MP" placed x (1, 0, 0) y (0, 1, 0) z (0, 0, 1) at (37.973, 25.493, 1.57) in component "PCB Component"
component "SOLDERJUMPER_ARROW_NOPASTE" placed x (0, 1, 0) y (-1, 0, 0) z (0, 0, 1) at (17.838, 34.465, 1.57) in component "PCB Component"
component "SOLDERJUMPER_ARROW_NOPASTE" placed x (0, 1, 0) y (-1, 0, 0) z (0, 0, 1) at (23.501, 34.496, 1.57) in component "PCB Component"
component "MOUNTINGHOLE_3.0_PLATED" placed x (1, 0, 0) y (0, 1, 0) z (0, 0, 1) at (4, 79.8, 1.57) in component "PCB Component"
component "MOUNTINGHOLE_3.0_PLATED" placed x (1, 0, 0) y (0, 1, 0) z (0, 0, 1) at (116.7, 79.8, 1.57) in component "PCB Component"
component "MOUNTINGHOLE_3.0_PLATED" placed x (1, 0, 0) y (0, 1, 0) z (0, 0, 1) at (116.7, -4, 1.57) in component "PCB Component"
component "MOUNTINGHOLE_3.0_PLATED" placed x (1, 0, 0) y (0, 1, 0) z (0, 0, 1) at (4, -4, 1.57) in component "PCB Component"
component "FIDUCIAL_1MM" placed x (1, 0, 0) y (0, 1, 0) z (0, 0, 1) at (36.3, 61.2, 1.57) in component "PCB Component"
component "FIDUCIAL_1MM" placed x (1, 0, 0) y (0, 1, 0) z (0, 0, 1) at (37.98, 32.45, 1.57) in component "PCB Component"
component "FIDUCIAL_1MM" placed x (1, 0, 0) y (0, 1, 0) z (0, 0, 1) at (118.63, 2.154, 1.57) in component "PCB Component"
component "FIDUCIAL_1MM" placed x (1, 0, 0) y (0, 1, 0) z (0, 0, 1) at (9.398, 71.755, 1.57) in component "PCB Component"
component "FIDUCIAL_1MM" placed x (1, 0, 0) y (0, 1, 0) z (0, 0, 1) at (7.239, 3.175, 1.57) in component "PCB Component"
component "FIDUCIAL_1MM" placed x (1, 0, 0) y (0, 1, 0) z (0, 0, 1) at (118.618, 74.041, 1.57) in component "PCB Component"
component "SOT23-5" placed x (0, -1, 0) y (1, 0, 0) z (0, 0, 1) at (23.5, 66.5, 1.57) in component "PCB Component"
component "SOT23-5" placed x (0, 1, 0) y (-1, 0, 0) z (0, 0, 1) at (41.4, 66.5, 1.57) in component "PCB Component"
component "SOT223-R" placed x (-1, 0, 0) y (0, -1, 0) z (0, 0, 1) at (18.4, 24.2, 1.57) in component "PCB Component"
component "4UCONN_20329" placed x (0, -1, 0) y (1, 0, 0) z (0, 0, 1) at (3.75, 29.6, 1.57) in component "PCB Component"
component "TSSOP20-5.3MMBODY" placed x (0, 1, 0) y (-1, 0, 0) z (0, 0, 1) at (46.101, 25.366, 1.57) in component "PCB Component"
component "RESONATOR-SMD" placed x (0, 1, 0) y (-1, 0, 0) z (0, 0, 1) at (52.186, 22.408, 1.57) in component "PCB Component"
component "RESPACK_4X0603" placed x (0, -1, 0) y (1, 0, 0) z (0, 0, 1) at (46.95, 47.1, 1.57) in component "PCB Component"
component "RESPACK_4X0603" placed x (0, -1, 0) y (1, 0, 0) z (0, 0, 1) at (46.95, 51.2, 1.57) in component "PCB Component"
component "RESPACK_4X0603" placed x (-1, 0, 0) y (0, -1, 0) z (0, 0, 1) at (35.4, 37.05, 1.57) in component "PCB Component"
component "RESPACK_4X0603" placed x (-1, 0, 0) y (0, -1, 0) z (0, 0, 1) at (39.5, 37.05, 1.57) in component "PCB Component"
component "RESPACK_4X0603" placed x (-1, 0, 0) y (0, -1, 0) z (0, 0, 1) at (27.2, 34.3, 1.57) in component "PCB Component"
component "RESPACK_4X0603" placed x (-1, 0, 0) y (0, -1, 0) z (0, 0, 1) at (31.3, 34.3, 1.57) in component "PCB Component"
component "RESPACK_4X0603" placed x (0, -1, 0) y (1, 0, 0) z (0, 0, 1) at (46.95, 55.3, 1.57) in component "PCB Component"
component "CHIPLED_0805_NOOUTLINE" placed x (1, 0, 0) y (0, 1, 0) z (0, 0, 1) at (1, 2.145, 1.57) in component "PCB Component"
component "CHIPLED_0805_NOOUTLINE" placed x (-1, 0, 0) y (0, -1, 0) z (0, 0, 1) at (1.1, 21.5, 1.57) in component "PCB Component"
component "CHIPLED_0805_NOOUTLINE" placed x (-1, 0, 0) y (0, -1, 0) z (0, 0, 1) at (1, 11.822, 1.57) in component "PCB Component"
component "INDUCTOR_5X5MM_NR5040_NOTHERMALS" placed x (1, 0, 0) y (0, 1, 0) z (0, 0, 1) at (41.5, 60.4, 1.57) in component "PCB Component"
component "SOD-123" placed x (-1, 0, 0) y (0, -1, 0) z (0, 0, 1) at (47.3, 59.2, 1.57) in component "PCB Component"
component "SMADIODE" placed x (0, 1, 0) y (-1, 0, 0) z (0, 0, 1) at (48.8, 64.1, 1.57) in component "PCB Component"
component "SOT23-WIDE" placed x (0, 1, 0) y (-1, 0, 0) z (0, 0, 1) at (7.268, 10.698, 1.57) in component "PCB Component"
component "TFTLCD-KD50G21-40NT-A1" placed x (-1, 0, 0) y (0, 1, 0) z (0, 0, -1) at (120.7, 0, 0) in component "PCB Component"
component "1X01_SMD_MASKHELD_2X2MM" placed x (1, 0, 0) y (0, 1, 0) z (0, 0, 1) at (1.6, 73.3, 1.57) in component "PCB Component"
component "1X01_SMD_MASKHELD_2X2MM" placed x (1, 0, 0) y (0, 1, 0) z (0, 0, 1) at (1.6, 64.9, 1.57) in component "PCB Component"
component "1X01_SMD_MASKHELD_2X2MM" placed x (1, 0, 0) y (0, 1, 0) z (0, 0, 1) at (1.6, 62.1, 1.57) in component "PCB Component"
component "1X01_SMD_MASKHELD_2X2MM" placed x (1, 0, 0) y (0, 1, 0) z (0, 0, 1) at (1.6, 67.7, 1.57) in component "PCB Component"
component "1X01_SMD_MASKHELD_2X2MM" placed x (1, 0, 0) y (0, 1, 0) z (0, 0, 1) at (1.6, 70.5, 1.57) in component "PCB Component"
component "1X01_SMD_MASKHELD_2X2MM" placed x (1, 0, 0) y (0, 1, 0) z (0, 0, 1) at (1.7, 37.2, 1.57) in component "PCB Component"
component "1X01_SMD_MASKHELD_2X2MM" placed x (1, 0, 0) y (0, 1, 0) z (0, 0, 1) at (1.7, 40, 1.57) in component "PCB Component"
component "SOLDERJUMPER_CLOSEDWIRE" placed x (1, 0, 0) y (0, 1, 0) z (0, 0, 1) at (41.91, 69.596, 1.57) in component "PCB Component"
component "SOLDERJUMPER_CLOSEDWIRE" placed x (1, 0, 0) y (0, 1, 0) z (0, 0, 1) at (37.846, 19.304, 1.57) in component "PCB Component"
component "SOD-323" placed x (-1, 0, 0) y (0, -1, 0) z (0, 0, 1) at (53.721, 67.691, 1.57) in component "PCB Component"
component "PANASONIC_C" placed x (-1, 0, 0) y (0, -1, 0) z (0, 0, 1) at (9.017, 37.338, 1.57) in component "PCB Component"
component "ADAFRUIT_TEXT_30MM" placed x (1, 0, 0) y (0, 1, 0) z (0, 0, 1) at (69.596, 22.606, 1.57) in component "PCB Component"
component "PCBFEAT-REV-056" placed x (1, 0, 0) y (0, 1, 0) z (0, 0, 1) at (101.1, 13.2, 1.57) in component "PCB Component"
hidden bodies 7 20 25
named bodies: "Board", "HDMI_MOLEX_47151-0001_DIMLAYER", "S-PQFP-G100", "0805-NO", "_0805MP", "SOLDERJUMPER_ARROW_NOPASTE", "MOUNTINGHOLE_3.0_PLATED", "FIDUCIAL_1MM", "SOT23-5", "SOT223-R", "4UCONN_20329", "TSSOP20-5.3MMBODY", "RESONATOR-SMD", "RESPACK_4X0603", "CHIPLED_0805_NOOUTLINE", "INDUCTOR_5X5MM_NR5040_NOTHERMALS", "SOD-123", "SMADIODE", "SOT23-WIDE", "TFTLCD-KD50G21-40NT-A1", "1X01_SMD_MASKHELD_2X2MM", "SOLDERJUMPER_CLOSEDWIRE", "SOD-323", "PANASONIC_C", "ADAFRUIT_TEXT_30MM", "PCBFEAT-REV-056"
